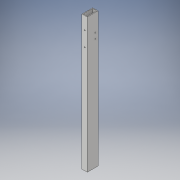
# Autodesk Inventor part: 2xtopPost
Saved by Autodesk Inventor 2018.2 (Build 222227000, 227)
## iProperties
Created: 2018-02-08
Part Number: 2xtopPost
Material: Generic
Document SubType Name: Modeling
Designer: steele
Density: 1 g/cm^3
Appearance: Default
Author: steele
Autodesk Inventor part; units mm, degrees
ref_plane "YZ Plane" through (0, 0, 0) normal (1, 0, 0) x (0, 1, 0)
ref_plane "XZ Plane" through (0, 0, 0) normal (0, 1, 0) x (-1, 0, 0)
ref_plane "XY Plane" through (0, 0, 0) normal (0, 0, 1) x (1, 0, 0)
sketch "Sketch1" plane through (0, 0, 0) normal (0, 1, 0) x (-1, 0, 0)
  line L0 (12.7, 25.4) -> (-12.7, 25.4)
  line L1 (-12.7, 25.4) -> (-12.7, -25.4)
  line L2 (-12.7, -25.4) -> (12.7, -25.4)
  line L3 (12.7, -25.4) -> (12.7, 25.4)
  line L4 (12.7, 25.4) -> (-12.7, -25.4) construction
  line L5 (-12.7, 25.4) -> (12.7, -25.4) construction
  line L6 (9.525, 22.225) -> (-9.525, 22.225)
  line L7 (-9.525, 22.225) -> (-9.525, -22.225)
  line L8 (-9.525, -22.225) -> (9.525, -22.225)
  line L9 (9.525, -22.225) -> (9.525, 22.225)
  line L10 (9.525, 22.225) -> (-9.525, -22.225) construction
  line L11 (-9.525, 22.225) -> (9.525, -22.225) construction
  point P0 (0, 0)
  dimension "d0" = 25.4
  dimension "d1" = 3.175
  dimension "d4" = 50.8
  dimension "d5" = 19.05
  constraints: 24 end point, 4 midpoint, 4 parallel, 2 horizontal, 2 perpendicular
  measures "d0" distance of L0.start L0.end
  measures "d1" distance between parallel lines of L6 L0
  measures "d4" distance of L2.end L0.start
  measures "d5" distance of L6.start L6.end
extrude "Extrusion1" add sketch "Sketch1" along normal blind 635
sketch "Sketch2" plane through (12.7, 0, -25.4) normal (0, 0, -1) x (-1, 0, 0)
  point P0 (12.7, 574.675)
hole "Hole1" at (0, 574.675, -25.4) direction (0, 0, 1) diameter 5.08 depth 3.175
sketch "Sketch3" plane through (-12.7, 0, 25.4) normal (0, 0, 1) x (1, 0, 0)
  point P0 (12.7, 574.675)
hole "Hole3" at (0, 574.675, 25.4) direction (0, 0, -1) diameter 5.08 depth 3.175
sketch "Sketch4" plane through (12.7, 0, -25.4) normal (0, 0, -1) x (-1, 0, 0)
  point P0 (12.7, 504.825)
hole "Hole5" at (0, 504.825, -25.4) direction (0, 0, 1) diameter 5.08 depth 3.175
sketch "Sketch5" plane through (-12.7, 0, 25.4) normal (0, 0, 1) x (1, 0, 0)
  point P0 (12.7, 504.825)
hole "Hole7" at (0, 504.825, 25.4) direction (0, 0, -1) diameter 5.08 depth 3.175
sketch "Sketch6" plane through (12.7, 0, 25.4) normal (1, 0, 0) x (0, 0, -1)
  point P0 (38.1, 552.45)
  point P1 (38.1, 527.05)
hole "Hole9" at (12.7, 552.45, -12.7) at (12.7, 527.05, -12.7) direction (-1, 0, 0) diameter 5.08 depth 3.175
sketch "Sketch7" plane through (-12.7, 0, -25.4) normal (-1, 0, 0) x (0, 0, 1)
  point P0 (12.7, 552.45)
  point P1 (12.7, 527.05)
hole "Hole11" at (-12.7, 552.45, -12.7) at (-12.7, 527.05, -12.7) direction (1, 0, 0) diameter 5.08 depth 3.175
body "Solid1"
